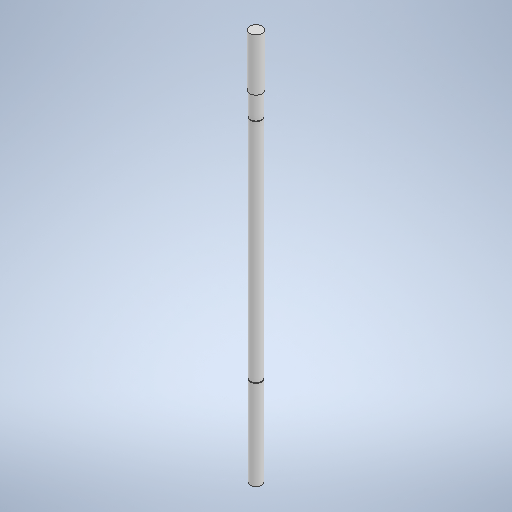
# Autodesk Inventor part: Вал
Saved by Autodesk Inventor 2025 (Build 290162010, 162A)
## iProperties
Created: 2024-04-09
Part Number: Вал
Material: Generic
Document SubType Name: Modeling
Designer: pokla
Density: 1 g/cm^3
Appearance: Default
Author: pokla
Autodesk Inventor part; units mm, degrees
ref_plane "YZ Plane" through (0, 0, 0) normal (1, 0, 0) x (0, 1, 0)
ref_plane "XZ Plane" through (0, 0, 0) normal (0, 1, 0) x (-1, 0, 0)
ref_plane "XY Plane" through (0, 0, 0) normal (0, 0, 1) x (1, 0, 0)
sketch "Sketch1" plane through (0, 0, 0) normal (1, 0, 0) x (0, 1, 0)
  line L0 (300, 0) -> (-300, 0)
  line L1 (-300, 0) -> (-300, -8.5)
  line L2 (-300, -8.5) -> (-163, -8.5)
  line L3 (300, -8.5) -> (300, 0)
  line L4 (185, -8.5) -> (185, -7.5)
  line L5 (185, -7.5) -> (184, -7.5)
  line L6 (184, -7.5) -> (184, -8.5)
  line L7 (-162, -7.5) -> (-163, -7.5)
  line L8 (-163, -7.5) -> (-163, -8.5)
  line L9 (-163, -8.5) -> (-162, -8.5) construction
  line L10 (-162, -8.5) -> (-162, -7.5)
  line L11 (220, -8.5) -> (300, -8.5) construction
  line L12 (300, -8.5) -> (220, -8.5) construction
  line L13 (220, -8.5) -> (220, -9.5)
  line L14 (220, -9.5) -> (300, -9.5)
  line L15 (300, -9.5) -> (300, -8.5)
  line L16 (184, -8.5) -> (185, -8.5) construction
  line L17 (185, -8.5) -> (220, -8.5)
  line L18 (-162, -8.5) -> (184, -8.5)
  line L19 (-163, -8.5) -> (-162, -8.5) construction
  point P0 (0, 0)
  point P1 (0, 0)
  point P2 (-163, -8.5)
  point P3 (-162, -8.5)
  dimension "d0" = 600
  dimension "d1" = 8.5
  dimension "d2" = 1
  dimension "d3" = 1
  dimension "d4" = 115
  dimension "d6" = 1
  dimension "d7" = 1
  dimension "d8" = 462
  dimension "d11" = 1
  dimension "d12" = 80
  constraints: 40 end point, 11 parallel, 10 perpendicular, 3 horizontal, 1 coincident, 1 midpoint, 1 point on line, 1 vertical
  measures "d0" distance of L3.start L1.end
  measures "d1" distance of L1.end L0.end
  measures "d2" distance of L4.start L4.end
  measures "d3" distance of L4.end L5.end
  measures "d4" distance between parallel lines of L3 L4
  measures "d6" distance of L9.end L7.start
  measures "d7" distance of L7.start L7.end
  measures "d8" distance between parallel lines of L3 L10
  measures "d11" distance of L12.end L13.end
  measures "d12" distance between parallel lines of L15 L13
revolve "Revolution1" add sketch "Sketch1" angle 360 about axis through (0, 300, 0) along (0, -1, 0)
equation "\"d6\" = d2"
equation "\"d7\" = d3"
body "Solid1"
